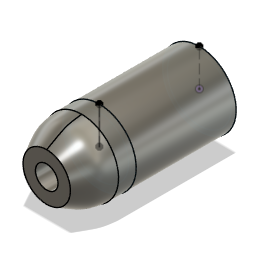
Lampa v12 (Autodesk Fusion 360 archive; units mm, degrees)
design "Suport Bec"
Autodesk Fusion 360 part; units mm, degrees
sketch "Sketch2" plane through (0, 0, 0) normal (0, 0, 1) x (1, 0, 0)
  circle A0 centre (0, 0) radius 14
  dimension "d1" = 28
  constraint coincident A0.centre origin
  measures "d1" diameter of A0
extrude "Extrude1" add sketch "Sketch2" along normal blind 38 makes body 1
sketch "Sketch3" plane through (0, 0, 38) normal (0, 0, 1) x (1, 0, 0)
  circle A0 centre (0, 0) radius 14
  circle A1 centre (0, 0) radius 7
  dimension "d4" = 14
  constraint coincident A0.centre A1.centre
  measures "d4" diameter of A1
extrude "Extrude2" cut sketch "Sketch3" against normal up to surface (38 mm away) contours A1 bodies 1
sketch "Sketch4" plane through (0, 0, 38) normal (0, 0, 1) x (1, 0, 0)
  circle A0 centre (0, 0) radius 7
  circle A1 centre (0, 0) radius 14
  circle A2 centre (0, 0) radius 11.15
  dimension "d7" = 22.3
  constraint coincident A0.centre A1.centre
  measures "d7" diameter of A2
extrude "Extrude3" cut sketch "Sketch4" against normal blind 18 contours A2 bodies 1
sketch "Sketch5" plane through (0, 0, 0) normal (0, 0, -1) x (-1, 0, 0)
  circle A0 centre (0, 0) radius 7
  circle A1 centre (0, 0) radius 14
  circle A2 centre (0, 0) radius 12.15
  dimension "d10" = 24.3
  constraint coincident A0.centre A1.centre
  measures "d10" diameter of A2
extrude "Extrude4" cut sketch "Sketch5" against normal blind 14.3 contours A2 bodies 1
copy_body "Body->Comp1" bodies 1 removing the originals makes body 2 in component "Soclu"
sketch "Sketch6" plane through (0, 0, 38) normal (0, 0, 1) x (1, 0, 0)
  circle A0 centre (0, 0) radius 11.15
  circle A1 centre (0, 0) radius 14
  line L0 (0, 0) -> (0, 14) construction
  line L1 (0, 0) -> (0, 14)
  constraint coincident A0.centre A1.centre
  constraint coincident A1 L0.end
  constraint vertical L0
sketch "Sketch7" plane through (0, 0, 0) normal (0, 0, -1) x (-1, 0, 0)
  circle A0 centre (0, 0) radius 12.15
  circle A1 centre (0, 0) radius 14
  line L0 (0, 0) -> (0, 14) construction
  constraint coincident A0.centre A1.centre
  constraint coincident A1 L0.end
  constraint vertical L0
ref_plane "WorkPlane1" through (0, 0, 0) normal (-1, 0, 0) x (0, -1, 0)
sketch "Sketch8" plane through (0, 0, 0) normal (-1, 0, 0) x (0, 0, 1)
  line L0 (38, -14) -> (38, 14)
  line L1 (0, -14) -> (0, 14)
  line L2 (38, 0) -> (58, 0) construction
  line L3 (58, 0) -> (58, 9)
  line L4 (38, 0) -> (44.7, 0)
  line L5 (44.7, 0) -> (44.7, 14)
  line L6 (44.7, 14) -> (38, 14)
  line L7 (38, 14) -> (38, 0)
  line L8 (38, 0) -> (58, 0)
  line L9 (58, 0) -> (58, 4.3)
  line L10 (58, 4.3) -> (38, 4.3)
  line L11 (38, 4.3) -> (38, 0)
  spline S0 degree 2 poles (58, 9) (50.5079, 13.2797) (44.7, 14) knots 0 0 0 1.435982 1.435982 1.435982 weights 1 3 1
  point P0 (38, 14)
  dimension "d13" = 20
  dimension "d14" = 9
  dimension "d15" = 6.7
  dimension "d16" = 4.3
  constraint midpoint L0 L2.start
  constraint perpendicular L0 L2
  constraint vertical L3
  constraint horizontal L4
  constraint vertical L5
  constraint horizontal L6
  constraint vertical L7
  constraint coincident L6 P0
  constraint horizontal L8
  constraint vertical L9
  constraint horizontal L10
  constraint vertical L11
  constraint coincident L3 L9.end
  measures "d13" distance of L2.start L2.end
  measures "d14" distance of L2.end L3.end
  measures "d15" distance of L5.end P0
  measures "d16" distance of L2 L10
revolve "Revolve1" add sketch "Sketch8" angle 360 about axis through (0, 0, 0) along (0, 0, -1) separate body contours L0 L5 L6 L7 L10 | L3 L5 L10 S0 makes body 3 in component "Soclu"
component "Soclu" placed x (1, 0, 0) y (0, 1, 0) z (0, 0, 1) at (0, 0, 0)
equation "d14 = 18 mm / 2"
equation "d16 = 8.6 mm / 2"
named bodies: "Soclu", "Cap_Soclu"

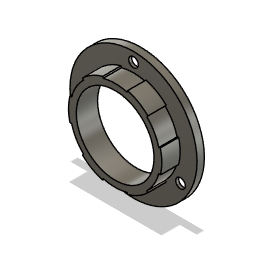
design "Adaptor Montare Suport Bec"
Autodesk Fusion 360 part; units mm, degrees
sketch "Sketch1" plane through (0, 0, 0) normal (0, 0, 1) x (1, 0, 0)
  circle A0 centre (0, 0) radius 21.65
  dimension "d1" = 43.3
  constraint coincident A0.centre origin
  measures "d1" diameter of A0
extrude "Extrude1" add sketch "Sketch1" along normal blind 2.5 makes body 1
sketch "Sketch2" plane through (0, 0, 0) normal (0, 0, -1) x (-1, 0, 0)
  circle A0 centre (0, 0) radius 21.65
  circle A1 centre (0, 0) radius 20.5
  dimension "d4" = 41
  constraint coincident A0.centre A1.centre
  measures "d4" diameter of A1
extrude "Extrude2" cut sketch "Sketch2" against normal blind 1.5 contours A1 bodies 1
sketch "Sketch3" plane through (0, 0, 2.5) normal (0, 0, 1) x (1, 0, 0)
  circle A0 centre (0, 0) radius 21.65
  circle A1 centre (0, 0) radius 15.35
  dimension "d7" = 30.7
  constraint concentric A0 A1
  measures "d7" diameter of A1
extrude "Extrude3" add sketch "Sketch3" along normal blind 6.25 contours A1 bodies 1
sketch "Sketch4" plane through (0, 0, 8.75) normal (0, 0, 1) x (1, 0, 0)
  circle A0 centre (0, 0) radius 15.35
  circle A1 centre (0, 0) radius 13.25
  dimension "d10" = 26.5
  constraint coincident A0.centre A1.centre
  measures "d10" diameter of A1
extrude "Extrude4" cut sketch "Sketch4" against normal up to surface (7.25 mm away) contours A1 bodies 1
sketch "Sketch5" plane through (0, 0, 2.5) normal (0, 0, 1) x (1, 0, 0)
  circle A0 centre (0, 0) radius 15.35
  circle A1 centre (0, 0) radius 21.65
  circle A2 centre (0, 0) radius 21.65
  line L0 (0, 0) -> (0, 21.65) construction
  line L1 (0, 15.35) -> (0, 21.65) construction
  circle A3 centre (0, 18.5) radius 1.65
  circle A4 centre (-16.0215, -9.25) radius 1.65
  circle A5 centre (16.0215, -9.25) radius 1.65
  dimension "d13" = 3.3
  dimension "d15" = 360
  constraint coincident A0.centre A1.centre
  constraint coincident A1 L0.end
  constraint vertical L0
  constraint coincident A0 L1.start
  constraint coincident L0 L1.start
  constraint midpoint L1 A3.centre
  measures "d13" diameter of A3
extrude "Extrude5" cut sketch "Sketch5" against normal up to surface (1 mm away) contours A3 | A4 | A5 bodies 1
sketch "Sketch6" plane through (0, 0, 8.75) normal (0, 0, 1) x (1, 0, 0)
  circle A0 centre (0, 0) radius 13.25
  circle A1 centre (0, 0) radius 15.35
  circle A2 centre (0, 0) radius 13.25
  circle A3 centre (0, 0) radius 21.65
  circle A4 centre (0, 18.5) radius 1.65
  circle A5 centre (0, 0) radius 15.35
  line L0 (0, 0) -> (0, 18.5) construction
  line L1 (0, 0) -> (0, -18.5) construction
  circle A6 centre (0, 0) radius 15.9 construction
  circle A7 centre (-16.0215, -9.25) radius 1.65
  arc A8 (0, 18.5) -> (-16.0215, -9.25) centre (0, 0) ccw construction
  arc A9 (0, 18.5) -> (-9.25, 16.0215) centre (0, 0) ccw construction
  line L2 (0, 0) -> (0, 18.5) construction
  line L3 (0, 0) -> (-9.25, 16.0215) construction
  arc A10 (-18.5, 0) -> (-16.0215, -9.25) centre (0, 0) ccw
  line L4 (0, 0) -> (-18.5, 0) construction
  line L5 (0, 0) -> (-16.0215, -9.25) construction
  arc A11 (-4.2302, 15.3269) -> (-11.1584, 11.3269) centre (0, 0) ccw
  line L6 (0, 0) -> (-4.2302, 15.3269) construction
  line L7 (0, 0) -> (-11.1584, 11.3269)
  line L8 (-4.2302, 15.3269) -> (-11.1584, 11.3269) construction
  line L9 (-11.1584, 11.3269) -> (-10.7724, 10.9351) construction
  line L10 (-4.2302, 15.3269) -> (-4.0839, 14.7968) construction
  line L11 (-4.2302, 15.3269) -> (-4.0839, 14.7968)
  dimension "d18" = 31.8
  dimension "d19" = 30
  dimension "d20" = 30
  dimension "d22" = 8
  constraint coincident A0.centre A1.centre
  constraint coincident A4.centre L0.end
  constraint parallel L0 L1
  constraint equal L0 L1
  constraint coincident A7.centre A8.end
  constraint coincident A6 A11.end
  constraint coincident A6 A11.start
  constraint perpendicular L3 L8
  constraint coincident L7 L9.end
  constraint coincident A5 L9.end
  constraint coincident L6 L10.end
  constraint coincident A1 L10.end
  measures "d18" diameter of A6
  measures "d19" angle of L2 L3
  measures "d20" angle of L4 L5
  measures "d22" distance of A11.start A11.end
extrude "Extrude6" add sketch "Sketch6" against normal up to surface (6.25 mm away) contours A1 A5 A11 L7 L11 bodies 1
pattern_circular "C-Pattern1" count 6 over 360 about axis through (0, 0, 1.75) along (0, 0, 1) of "Extrude6"
copy_body "Body->Comp1" bodies 1 removing the originals makes body 2 in component "Montare Soclu"
ref_plane "WorkPlane1" through (0, 0, -5.5) normal (0, 0, -1) x (-1, 0, 0)
sketch "Sketch7" plane through (0, 0, -5.5) normal (0, 0, -1) x (-1, 0, 0)
  circle A0 centre (0, 18.5) radius 1.65
  circle A1 centre (16.0215, -9.25) radius 1.65
  circle A2 centre (-16.0215, -9.25) radius 1.65
  circle A3 centre (0, 0) radius 13.25
  circle A4 centre (0, 0) radius 20.5
  circle A5 centre (0, 0) radius 21.65
  line L0 (-11.1584, 11.3269) -> (-10.7724, 10.9351)
  arc A6 (-10.7724, 10.9351) -> (-14.8563, 3.8616) centre (0, 0) ccw
  line L1 (-14.8563, 3.8616) -> (-15.3886, 4)
  arc A7 (-15.3886, 4) -> (-15.3886, -4) centre (0, 0) ccw
  line L2 (-15.3886, -4) -> (-14.8563, -3.8616)
  arc A8 (-14.8563, -3.8616) -> (-10.7724, -10.9351) centre (0, 0) ccw
  line L3 (-10.7724, -10.9351) -> (-11.1584, -11.3269)
  arc A9 (-11.1584, -11.3269) -> (-4.2302, -15.3269) centre (0, 0) ccw
  line L4 (-4.2302, -15.3269) -> (-4.0839, -14.7968)
  arc A10 (-4.0839, -14.7968) -> (4.0839, -14.7968) centre (0, 0) ccw
  line L5 (4.0839, -14.7968) -> (4.2302, -15.3269)
  arc A11 (4.2302, -15.3269) -> (11.1584, -11.3269) centre (0, 0) ccw
  line L6 (11.1584, -11.3269) -> (10.7724, -10.9351)
  arc A12 (10.7724, -10.9351) -> (14.8563, -3.8616) centre (0, 0) ccw
  line L7 (14.8563, -3.8616) -> (15.3886, -4)
  arc A13 (15.3886, -4) -> (15.3886, 4) centre (0, 0) ccw
  line L8 (15.3886, 4) -> (14.8563, 3.8616)
  arc A14 (14.8563, 3.8616) -> (10.7724, 10.9351) centre (0, 0) ccw
  line L9 (10.7724, 10.9351) -> (11.1584, 11.3269)
  arc A15 (11.1584, 11.3269) -> (4.2302, 15.3269) centre (0, 0) ccw
  line L10 (4.2302, 15.3269) -> (4.0839, 14.7968)
  arc A16 (4.0839, 14.7968) -> (-4.0839, 14.7968) centre (0, 0) ccw
  line L11 (-4.0839, 14.7968) -> (-4.2302, 15.3269)
  arc A17 (-4.2302, 15.3269) -> (-11.1584, 11.3269) centre (0, 0) ccw
  circle A18 centre (0, 18.5) radius 1.65
  circle A19 centre (16.0215, -9.25) radius 1.65
  circle A20 centre (-16.0215, -9.25) radius 1.65
  circle A21 centre (0, 0) radius 21.65
extrude "Extrude7" add sketch "Sketch7" along normal blind 3.5 separate body contours A4 | A5 A21 makes body 3
move_face "OffsetFaces1" offset -0.2 24 faces at (-3.4159, 14.9651, -6.6667) (4.8758, 15.1339, -6.6667) (-6.7556, 14.3935, -7.8333) (-11.7093, 9.9254, -7.8333) (12.9357, 8.2637, -7.8333) (15.5443, -3.3444, -7.8333) (14.6681, -4.5243, -6.6667) (8.5263, -13.4206, -7.8333) (-0.6887, -15.3345, -7.8333) (-10.6685, -11.7896, -7.8333) (-11.2522, -10.4408, -6.6667) (-15.5443, -3.3444, -6.6667) (-4.1814, 15.1502, -6.6667) (4.1327, 14.9735, -6.6667) (11.0298, 11.1963, -6.6667) (15.0338, 3.9078, -6.6667) (15.2112, -3.9539, -6.6667) (10.9011, -11.0657, -6.6667) (4.1814, -15.1502, -6.6667) (-4.1327, -14.9735, -6.6667) (-11.0298, -11.1963, -6.6667) (-15.0338, -3.9078, -6.6667) (-15.2112, 3.9539, -6.6667) (-10.9011, 11.0657, -6.6667) on bodies 3
component "Montare Soclu" placed x (1, 0, 0) y (0, 1, 0) z (0, 0, 1) at (0, 0, 0)
hidden bodies 3
named bodies: "Montare Soclu", "Test Soclu"

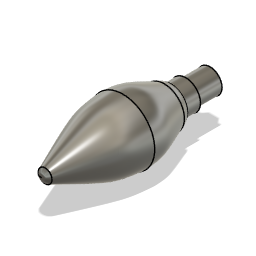
design "Bec E14"
Autodesk Fusion 360 part; units mm, degrees
sketch "Sketch2" plane through (0, 0, 0) normal (0, 1, 0) x (1, 0, 0)
  line L0 (0, 0) -> (0, -100)
  line L1 (0, -25) -> (-9.5, -25) construction
  line L2 (0, -25) -> (-8.5, -25)
  line L3 (-8.5, -25) -> (-8.5, -16.5)
  line L4 (-8.5, -16.5) -> (0, -16.5)
  line L5 (0, -16.5) -> (0, -25)
  line L6 (0, -16.5) -> (-7, -16.5)
  line L7 (-7, -16.5) -> (-7, -2.5)
  line L8 (-7, -2.5) -> (0, -2.5)
  line L9 (0, -2.5) -> (0, -16.5)
  line L10 (-8.5, -25) -> (-9.5, -25)
  line L11 (49.3295, 0) -> (-49.3295, 0) construction
  line L12 (-5, -2.5) -> (-3, 0)
  line L13 (0, -53) -> (-18.5, -53)
  line L14 (0, 0) -> (-3, 0)
  line L15 (0, -98) -> (-4, -98)
  spline S0 degree 2 poles (0, -100) (-2, -100) (-4, -98) knots 0 0 0 0.46731 0.46731 0.46731 weights 1 3 1
  spline S1 degree 2 poles (-4, -98) (-17.25, -67.629) (-18.5, -53) knots 0 0 0 4.756075 4.756075 4.756075 weights 1 3 1
  line L16 (0, -29) -> (-11.7087, -29)
  spline S2 degree 2 poles (-18.5, -53) (-18, -44) (-11.7087, -29) knots 0 0 0 2.512547 2.512547 2.512547 weights 1 3 1
  spline S3 degree 2 poles (-9.5, -25) (-10.4138, -25.5646) (-11.7087, -29) knots 0 0 0 0.464015 0.464015 0.464015 weights 1 2.333333 1
  point P0 (0, -25)
  point P1 (-8.5, -25)
  point P2 (-5, -2.5)
  point P3 (-3, 0)
  point P4 (0, -53)
  point P5 (0, -98)
  point P6 (0, -29)
  dimension "d1" = 100
  dimension "d2" = 25
  dimension "d3" = 9.5
  dimension "d4" = 8.5
  dimension "d5" = 14
  dimension "d6" = 7
  dimension "d7" = 5
  dimension "d8" = 3
  dimension "d9" = 28
  dimension "d10" = 18.5
  dimension "d14" = 2
  dimension "d15" = 4
  dimension "d18" = 4
  constraint coincident L0.start L14.start
  constraint vertical L0
  constraint coincident L0 P0
  constraint coincident P0 L1.start
  constraint perpendicular L0 L1
  constraint coincident L1 P1
  constraint horizontal L2
  constraint vertical L3
  constraint horizontal L4
  constraint vertical L5
  constraint equal L3 L4
  constraint coincident P1 L3
  constraint horizontal L6
  constraint vertical L7
  constraint horizontal L8
  constraint vertical L9
  constraint coincident P1 L2.end
  constraint coincident L8 P2
  constraint perpendicular L0 L11
  constraint midpoint L0.start L11
  constraint coincident L11 P3
  constraint coincident P2 L12.start
  constraint coincident P3 L12.end
  constraint coincident L0 P4
  constraint coincident P4 L13.start
  constraint perpendicular L0 L13
  constraint coincident L0 P5
  constraint coincident P5 L15.start
  constraint perpendicular L0 L15
  constraint coincident L0 P6
  constraint coincident P6 L16.start
  constraint perpendicular L0 L16
  measures "d1" distance of L0.start L0.end
  measures "d2" distance of L0.start L1.start
  measures "d3" distance of P0 L1.end
  measures "d4" distance of L0 P1
  measures "d5" distance of L6.end L7.end
  measures "d6" distance of L7.end L8.end
  measures "d7" distance of L0 P2
  measures "d8" distance of L0.start P3
  measures "d9" distance of P0 P4
  measures "d10" distance of P4 L13.end
  measures "d14" distance of L0.end P5
  measures "d15" distance of P5 L15.end
  measures "d18" distance of P0 P6
revolve "Revolve1" add sketch "Sketch2" angle 360 about axis through (0, 0, 0) along (0, 0, 1) makes body 1
copy_body "Body->Comp1" bodies 1 removing the originals makes body 2 in component "Bec E14"
component "Bec E14" placed x (1, 0, 0) y (0, 1, 0) z (0, 0, 1) at (0, 0, 0)
equation "d3 = ( 19 / 2 ) * 1 mm"
equation "d4 = ( 17 / 2 ) * 1 mm"
equation "d10 = ( 37 / 2 ) * 1 mm"
named bodies: "Bec E14"
